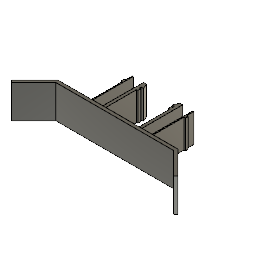
brade1_old (Autodesk Fusion 360 design; units mm, degrees)
Autodesk Fusion 360 part; units mm, degrees
sketch "スケッチ1" plane through (0, 0, 0) normal (0, 0, 1) x (1, 0, 0)
  line L0 (-40.0294, 0) -> (-27.2294, 0)
  line L1 (-27.2294, 0) -> (-27.2294, -2.8335)
  line L2 (-27.2294, -2.8335) -> (-40.0294, -2.8335)
  line L3 (-40.0294, -2.8335) -> (-40.0294, 0)
  line L4 (-40.0294, 0) -> (-39.0294, 0)
  line L5 (-39.0294, 0) -> (-39.0294, 39.9696)
  line L6 (-39.0294, 39.9696) -> (-40.0294, 39.9696)
  line L7 (-40.0294, 39.9696) -> (-40.0294, 0)
  line L8 (-27.2294, 0) -> (-28.3294, 0)
  line L9 (-28.3294, 0) -> (-28.3294, 40)
  line L10 (-28.3294, 40) -> (-27.2294, 40)
  line L11 (-27.2294, 40) -> (-27.2294, 0)
  line L12 (-27.2294, 0) -> (2.7706, 0)
  line L13 (2.7706, 0) -> (2.7706, -2.9213)
  line L14 (2.7706, -2.9213) -> (-27.2294, -2.9213)
  line L15 (-27.2294, -2.9213) -> (-27.2294, 0)
  line L16 (-12.2294, 0) -> (-12.2294, -2.9213)
  line L17 (2.7706, 0) -> (2.7706, -2.8335)
  line L18 (15.5706, 0) -> (2.7706, 0)
  line L19 (15.5706, 39.9696) -> (15.5706, 0)
  line L20 (3.8706, 0) -> (3.8706, 40)
  line L21 (14.5706, 39.9696) -> (15.5706, 39.9696)
  line L22 (15.5706, 0) -> (14.5706, 0)
  line L23 (14.5706, 0) -> (14.5706, 39.9696)
  line L24 (15.5706, -2.8335) -> (15.5706, 0)
  line L25 (2.7706, -2.9213) -> (2.7706, 0)
  line L26 (2.7706, 40) -> (2.7706, 0)
  line L27 (2.7706, 0) -> (3.8706, 0)
  line L28 (3.8706, 40) -> (2.7706, 40)
  line L29 (2.7706, -2.8335) -> (15.5706, -2.8335)
  line L30 (-27.2294, 40) -> (-25, 35)
  line L31 (-25, 35) -> (-27.2294, 35)
  line L32 (3.8706, 40) -> (2.7706, 40)
  line L33 (0.5411, 35) -> (2.7706, 35)
  line L34 (2.7706, 40) -> (0.5411, 35)
  dimension "d1" = 12.8
  dimension "d2" = 1
  dimension "d3" = 1.1
  dimension "d4" = 30
  constraint horizontal L0
  constraint vertical L1
  constraint horizontal L2
  constraint vertical L3
  constraint horizontal L4
  constraint vertical L5
  constraint horizontal L6
  constraint vertical L7
  constraint horizontal L8
  constraint vertical L9
  constraint horizontal L10
  constraint vertical L11
  constraint horizontal L12
  constraint vertical L13
  constraint horizontal L14
  constraint vertical L15
  constraint midpoint L12 L16.start
  constraint midpoint L14 L16.end
  constraint symmetric L0.start L16 L18.start
  constraint symmetric L0.end L16 L12.end
  constraint symmetric L1.end L16 L17.end
  constraint symmetric L2.end L16 L24.start
  constraint symmetric L4.end L16 L22.end
  constraint symmetric L5.end L16 L21.start
  constraint symmetric L6.end L16 L19.start
  constraint symmetric L8.end L16 L20.start
  constraint symmetric L9.end L16 L20.end
  constraint symmetric L10.end L16 L26.start
  constraint symmetric L14.end L16 L13.end
  constraint coincident L11 L31.end
  constraint perpendicular L11 L31
  constraint symmetric L16 L30.end L33.start
  constraint symmetric L16 L31.end L33.end
  measures "d1" distance of L0.start L0.end
  measures "d2" distance of L0.start L4.end
  measures "d3" distance of L0.end L8.end
  measures "d4" distance of L0.end L12.end
sketch "スケッチ2" plane through (0, 0, 0) normal (0, 0, 1) x (1, 0, 0)
  line L0 (-40, 34.6932) -> (-40, 33.4932)
  line L1 (-40, 33.4932) -> (-41.2402, 33.4932)
  line L2 (-41.2402, 33.4932) -> (-41.2402, 30.9431)
  line L3 (-41.2402, 30.9431) -> (-40, 30.9431)
  line L4 (-40, 30.9431) -> (-40, 33.4932)
  line L5 (-26, 34.6932) -> (-26, 33.4932)
  line L6 (-27.2402, 33.4932) -> (-27.2402, 30.9431)
  line L7 (-26, 30.9431) -> (-26, 33.4932)
  line L8 (-26, 33.4932) -> (-27.2402, 33.4932)
  line L9 (-27.2402, 30.9431) -> (-26, 30.9431)
  line L10 (-40, 33.4932) -> (-41.2402, 33.4932)
  line L11 (-40, 30.9431) -> (-40, 33.4932)
  line L12 (-41.2402, 33.4932) -> (-41.2402, 30.9431)
  line L13 (-41.2402, 30.9431) -> (-40, 30.9431)
  line L14 (-27.2402, 33.4932) -> (-27.2402, 30.9431)
  line L15 (-26, 33.4932) -> (-27.2402, 33.4932)
  line L16 (-27.2402, 30.9431) -> (-26, 30.9431)
  line L17 (-26, 34.6932) -> (-26, 33.4932)
  line L18 (-26, 30.9431) -> (-26, 33.4932)
  line L19 (-40, 34.6932) -> (-40, 33.4932)
  line L20 (-12.2294, 0) -> (-12.2294, -2.9213)
  line L21 (2.7813, 33.4932) -> (2.7813, 30.9431)
  line L22 (15.5411, 30.9431) -> (15.5411, 33.4932)
  line L23 (16.7813, 33.4932) -> (16.7813, 30.9431)
  line L24 (1.5411, 34.6932) -> (1.5411, 33.4932)
  line L25 (1.5411, 30.9431) -> (1.5411, 33.4932)
  line L26 (2.7813, 33.4932) -> (2.7813, 30.9431)
  line L27 (15.5411, 33.4932) -> (16.7813, 33.4932)
  line L28 (1.5411, 34.6932) -> (1.5411, 33.4932)
  line L29 (2.7813, 30.9431) -> (1.5411, 30.9431)
  line L30 (2.7813, 30.9431) -> (1.5411, 30.9431)
  line L31 (1.5411, 33.4932) -> (2.7813, 33.4932)
  line L32 (1.5411, 33.4932) -> (2.7813, 33.4932)
  line L33 (15.5411, 34.6932) -> (15.5411, 33.4932)
  line L34 (15.5411, 33.4932) -> (16.7813, 33.4932)
  line L35 (16.7813, 33.4932) -> (16.7813, 30.9431)
  line L36 (16.7813, 30.9431) -> (15.5411, 30.9431)
  line L37 (16.7813, 30.9431) -> (15.5411, 30.9431)
  line L38 (1.5411, 30.9431) -> (1.5411, 33.4932)
  line L39 (15.5411, 34.6932) -> (15.5411, 33.4932)
  line L40 (15.5411, 30.9431) -> (15.5411, 33.4932)
  dimension "d8" = 1.2
  dimension "d9" = 1.2
  dimension "d10" = 1.2
  dimension "d11" = 1.2
  constraint vertical L0
  constraint horizontal L1
  constraint vertical L2
  constraint horizontal L3
  constraint vertical L4
  constraint vertical L5
  constraint horizontal L8
  constraint vertical L6
  constraint horizontal L9
  constraint vertical L7
  constraint vertical L19
  constraint horizontal L10
  constraint vertical L12
  constraint horizontal L13
  constraint vertical L11
  constraint vertical L17
  constraint horizontal L15
  constraint vertical L14
  constraint horizontal L16
  constraint vertical L18
  constraint symmetric L0.start L20 L33.start
  constraint symmetric L0.end L20 L22.end
  constraint symmetric L1.end L20 L23.start
  constraint symmetric L2.end L20 L23.end
  constraint symmetric L3.end L20 L22.start
  constraint symmetric L5.end L20 L24.end
  constraint symmetric L5.start L20 L24.start
  constraint symmetric L6.start L20 L21.start
  constraint symmetric L6.end L20 L21.end
  constraint symmetric L7.start L20 L25.start
  measures "d8" distance of L0.start L0.end
  measures "d9" distance of L5.end L5.start
  measures "d10" distance of L0.end L0.start
  measures "d11" distance of L5.end L5.start
extrude "押し出し1" add sketch "スケッチ1" sketch "スケッチ2" along normal blind 25.8 of sketch 2
move_face "面をオフセット1" offset 1.5 1 faces at (-28.3294, 26.6667, 17.2)
move_face "面をオフセット2" offset 1.5 1 faces at (3.8706, 26.6667, 17.2)
sketch "スケッチ3" plane through (0, 0, 0) normal (0, 0, 1) x (1, 0, 0)
  line L0 (-22.2393, 22.0314) -> (-2.2393, 22.0314)
  line L1 (-2.2393, 22.0314) -> (-2.2393, 2.0314)
  line L2 (-2.2393, 2.0314) -> (-22.2393, 2.0314)
  line L3 (-22.2393, 2.0314) -> (-22.2393, 22.0314)
  line L4 (-29, 25) -> (4, 25)
  line L5 (4, 25) -> (4, -2)
  line L6 (4, -2) -> (-29, -2)
  line L7 (-29, -2) -> (-29, 25)
  dimension "d16" = 20
  dimension "d17" = 20
  constraint horizontal L0
  constraint vertical L1
  constraint horizontal L2
  constraint vertical L3
  constraint horizontal L4
  constraint vertical L5
  constraint horizontal L6
  constraint vertical L7
  measures "d16" distance of L0.start L0.end
  measures "d17" distance of L0.start L2.end
extrude "押し出し2" add sketch "スケッチ3" along normal blind 3
sketch "スケッチ4" plane through (0, 0, 0) normal (0, 0, 1) x (1, 0, 0)
  line L0 (-12, -2) -> (-67, -2)
  line L1 (-67, -2) -> (-67, -4)
  line L2 (-67, -4) -> (-12, -4)
  line L3 (-12, -4) -> (-12, -2)
  line L4 (-67, -2) -> (-65, -4)
  line L5 (-65, -4) -> (-85, -24)
  line L6 (-85, -24) -> (-87, -22)
  line L7 (-87, -22) -> (-67, -2)
  line L8 (61, -24) -> (63, -22)
  line L9 (41, -4) -> (61, -24)
  line L10 (-12, -2) -> (43, -2)
  line L11 (43, -2) -> (41, -4)
  line L12 (63, -22) -> (43, -2)
  line L13 (43, -2) -> (43, -4)
  line L14 (43, -4) -> (-12, -4)
  point P0 (-24, 0)
  constraint horizontal L0
  constraint vertical L1
  constraint horizontal L2
  constraint vertical L3
  constraint perpendicular L4 L5
  constraint parallel L4 L6
  constraint parallel L5 L7
  constraint coincident L2 L4.end
  constraint symmetric origin L3 P0
  constraint symmetric L0.start L3 L10.start
  constraint symmetric L0.end L3 L10.end
  constraint symmetric L1.end L3 L13.end
  constraint symmetric L2.end L3 L14.end
  constraint symmetric L3 L4.end L9.start
  constraint symmetric L3 L5.end L8.start
  constraint symmetric L3 L6.end L8.end
extrude "押し出し3" add sketch "スケッチ4" along normal blind 30
move_face "面をオフセット3" offset 1 1 faces at (33.8569, -2, 18.6)
